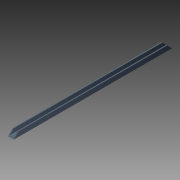
# Autodesk Inventor part: c-channel template
Saved by Autodesk Inventor 2012 (Build 160160000, 160)
## iProperties
Created: 2012-01-14
Part Number: c-channel template
Material: Aluminum-6061
Document SubType Name: Modeling
Designer: Antonella Wilby
Mass: 58.2867 g
Surface Area: 291.028 cm^2
Volume: 21.508 cm^3
Density: 2.71 g/cm^3
Author: Antonella Wilby
Autodesk Inventor part; units mm, degrees
ref_plane "YZ Plane" through (0, 0, 0) normal (1, 0, 0) x (0, 1, 0)
ref_plane "XZ Plane" through (0, 0, 0) normal (0, 1, 0) x (-1, 0, 0)
ref_plane "XY Plane" through (0, 0, 0) normal (0, 0, 1) x (1, 0, 0)
sketch "Sketch1" plane through (0, 0, 0) normal (0, 0, 1) x (1, 0, 0)
  line L0 (-6.6675, 0) -> (6.6675, 0) projected
  line L1 (0, -6.35) -> (0, 4.7625) projected
  line L2 (-3.175, 3.175) -> (-3.175, -3.175)
  line L3 (-3.175, -3.175) -> (3.175, -3.175)
  line L4 (3.175, -3.175) -> (3.175, 3.175)
  line L5 (4.7625, 3.175) -> (4.7625, -4.7625)
  line L6 (4.7625, -4.7625) -> (-4.7625, -4.7625)
  line L7 (-4.7625, -4.7625) -> (-4.7625, 3.175)
  line L8 (-3.175, 3.175) -> (-4.7625, 3.175)
  line L9 (3.175, 3.175) -> (4.7625, 3.175)
  point P0 (0, 0)
  point P1 (0, -3.175)
  point P2 (-3.175, 0)
  dimension "d0" = 1.5875
  dimension "d1" = 6.35
  dimension "d2" = 6.35
  constraints: 16 end point, 4 perpendicular, 3 parallel, 2 midpoint, 1 collinear, 1 horizontal alignment, 1 vertical alignment, 2 other
  measures "d0" distance between parallel lines of L4 L5
  measures "d1" distance between parallel lines of L2 L4
  measures "d2" distance between parallel lines of L8 L3
extrude "Extrusion1" add sketch "Sketch1" along normal mid plane 257.175 contours L7 L8 L2 L0 | L0 L2 L3 L1 L6 L7 | L1 L3 L4 L0 L5 L6 | L4 L9 L5 L0
sketch "Sketch2" plane through (4.7625, -4.7625, 128.5875) normal (1, 0, 0) x (0, 0, -1)
  line L0 (0, 7.9375) -> (0, 0) projected
  line L1 (0, 0) -> (257.175, 0) projected
  line L2 (0, 7.9375) -> (257.175, 7.9375) projected
  line L3 (0, 0) -> (7.9375, 7.9375)
  line L4 (7.9375, 7.9375) -> (0, 7.9375)
  line L5 (0, 7.9375) -> (0, 0)
  line L6 (128.5875, 7.9375) -> (128.5875, 0) construction
  line L7 (257.175, 7.9375) -> (257.175, 0)
  line L8 (257.175, 0) -> (249.2375, 7.9375)
  line L9 (257.175, 7.9375) -> (249.2375, 7.9375)
  line L10 (7.9375, 7.9375) -> (0, 7.9375)
  point P0 (128.5875, 4.7625)
  dimension "d5" = 45
  constraints: 16 end point, 3 symmetric about line, 2 midpoint, 1 collinear, 1 point on line
  measures "d5" angle of L5 L3
extrude "Extrusion2" cut sketch "Sketch2" against normal through all contours L2 L3 L0 | L8 L2 L7
sketch "Sketch3" plane through (-4.7625, -4.7625, 128.5875) normal (0, -1, 0) x (1, 0, 0)
  line L0 (0, 0) -> (0, -257.175) projected
  line L1 (9.525, 0) -> (9.525, -257.175) projected
  circle A0 centre (4.7625, -244.872) radius 1.5875
  circle A1 centre (4.7625, -194.072) radius 1.5875
  line L2 (0, -128.5875) -> (9.525, -128.5875) construction
  circle A2 centre (4.7625, -12.303) radius 1.5875
  circle A3 centre (4.7625, -63.103) radius 1.5875
  point P0 (4.7625, -128.5875)
  dimension "d8" = 3.175
  dimension "d9" = 50.8
  constraints: 4 centre point, 2 end point, 2 midpoint, 2 symmetric about line, 1 equal radius, 2 other
  measures "d8" diameter of A0
  measures "d9" distance of A1.centre A0.centre
extrude "Extrusion3" add sketch "Sketch3" along normal blind 1.5875
body "Solid1"
